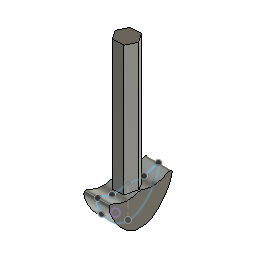
horse_support (Autodesk Fusion 360 design; units mm, degrees)
part number: 2026-05-20-21-49-29-160
Autodesk Fusion 360 part; units mm, degrees
derive "DerivedContext1"
sketch "Sketch1" plane through (0, 0, 0) normal (1, 0, 0) x (0, 1, 0)
  line L0 (-161.6595, 88.3093) -> (-161.6595, 78.1224)
  spline S0 degree 5 poles (-161.6595, 88.3093) (-161.5029, 88.2799) (-161.1728, 88.2083) (-160.6272, 88.0626) (-159.8017, 87.8168) (-158.6304, 87.5525) (-157.3592, 87.4678) (-156.0437, 87.6541) (-154.7574, 88.0873) (-153.5882, 88.6143) (-152.6243, 89.0285) (-151.9436, 89.1235) (-151.601, 88.7551) (-151.6157, 87.9035) (-151.9774, 86.6432) (-152.6539, 85.1075) (-153.5977, 83.4578) (-154.7519, 81.8484) (-156.0558, 80.4054) (-157.4494, 79.2317) (-158.8779, 78.4066) (-160.0123, 78.0714) (-160.8446, 78.0183) (-161.3895, 78.0728) (-161.6595, 78.1224) knots 0 0 0 0 0 0 0.05 0.1 0.15 0.2 0.25 0.3 0.35 0.4 0.45 0.5 0.55 0.6 0.65 0.7 0.75 0.8 0.85 0.9 0.95 1 1 1 1 1 1
  line L1 (-165.3917, 89.0107) -> (-157.9274, 87.6079)
  line L2 (-157.7822, 77.4094) -> (-165.5368, 78.8354)
  spline S1 degree 5 poles (-161.6595, 88.3093) (-161.8161, 88.2799) (-162.1462, 88.2083) (-162.6919, 88.0626) (-163.5173, 87.8168) (-164.6886, 87.5525) (-165.9599, 87.4678) (-167.2754, 87.6541) (-168.5616, 88.0873) (-169.7309, 88.6143) (-170.6948, 89.0285) (-171.3755, 89.1235) (-171.718, 88.7551) (-171.7033, 87.9035) (-171.3417, 86.6432) (-170.6652, 85.1075) (-169.7214, 83.4578) (-168.5671, 81.8484) (-167.2632, 80.4054) (-165.8696, 79.2317) (-164.4412, 78.4066) (-163.3067, 78.0714) (-162.4745, 78.0183) (-161.9295, 78.0728) (-161.6595, 78.1224) knots 0 0 0 0 0 0 0.05 0.1 0.15 0.2 0.25 0.3 0.35 0.4 0.45 0.5 0.55 0.6 0.65 0.7 0.75 0.8 0.85 0.9 0.95 1 1 1 1 1 1
  line L3 (-157.9274, 89.0107) -> (-165.3917, 87.6079)
  line L4 (-165.5368, 77.4094) -> (-157.7822, 78.8354)
  point P0 (-156.5652, 87.6135)
  point P1 (-152, 89)
  point P2 (-153.319, 84)
  point P3 (-166.7538, 87.6135)
  point P4 (-171.319, 89)
  point P5 (-170, 84)
  constraint vertical L0
  constraint coincident L0 S0.end
  constraint midpoint L0.start L1
  constraint midpoint L0.end L2
  constraint symmetric P0 L0 P3
  constraint symmetric P1 L0 P4
  constraint symmetric P2 L0 P5
  constraint symmetric L0 S0.start S1.start
  constraint symmetric L0 S0.end S1.end
  constraint symmetric L0 L1.start L3.start
  constraint symmetric L0 L1.end L3.end
  constraint symmetric L0 L2.start L4.start
  constraint symmetric L0 L2.end L4.end
extrude "Extrude1" add sketch "Sketch1" along normal mid plane 8
sketch "Sketch2" plane through (-4, 0, 0) normal (-1, 0, 0) x (0, -1, 0)
  spline S0 degree 5 poles (161.6595, 78.1224) (161.9295, 78.0728) (162.4745, 78.0183) (163.3067, 78.0714) (164.4412, 78.4066) (165.8696, 79.2317) (167.2632, 80.4054) (168.5671, 81.8484) (169.7214, 83.4578) (170.6652, 85.1075) (171.3417, 86.6432) (171.7033, 87.9035) (171.718, 88.7551) (171.3755, 89.1235) (170.6948, 89.0285) (169.7309, 88.6143) (168.5616, 88.0873) (167.2754, 87.6541) (165.9599, 87.4678) (164.6886, 87.5525) (163.5173, 87.8168) (162.6919, 88.0626) (162.1462, 88.2083) (161.8161, 88.2799) (161.6595, 88.3093) knots -1 -1 -1 -1 -1 -1 -0.95 -0.9 -0.85 -0.8 -0.75 -0.7 -0.65 -0.6 -0.55 -0.5 -0.45 -0.4 -0.35 -0.3 -0.25 -0.2 -0.15 -0.1 -0.05 0 0 0 0 0 0
  spline S1 degree 5 poles (161.6595, 88.3093) (161.5029, 88.2799) (161.1728, 88.2083) (160.6272, 88.0626) (159.8017, 87.8168) (158.6304, 87.5525) (157.3592, 87.4678) (156.0437, 87.6541) (154.7574, 88.0873) (153.5882, 88.6143) (152.6243, 89.0285) (151.9436, 89.1235) (151.601, 88.7551) (151.6157, 87.9035) (151.9774, 86.6432) (152.6539, 85.1075) (153.5977, 83.4578) (154.7519, 81.8484) (156.0558, 80.4054) (157.4494, 79.2317) (158.8779, 78.4066) (160.0123, 78.0714) (160.8446, 78.0183) (161.3895, 78.0728) (161.6595, 78.1224) knots 0 0 0 0 0 0 0.05 0.1 0.15 0.2 0.25 0.3 0.35 0.4 0.45 0.5 0.55 0.6 0.65 0.7 0.75 0.8 0.85 0.9 0.95 1 1 1 1 1 1
ref_plane "WorkPlane1" through (-4, -160.339, 88.8588) normal (0, 0, 1) x (-1, 0, 0)
sketch "Sketch3" plane through (0, 0, 88.8588) normal (0, 0, 1) x (1, 0, 0)
  line L0 (1.9423, -164.9116) -> (3.4927, -161.7737)
  line L1 (3.4927, -161.7737) -> (1.5503, -158.8621)
  line L2 (1.5503, -158.8621) -> (-1.9423, -159.0884)
  line L3 (-1.9423, -159.0884) -> (-3.4927, -162.2263)
  line L4 (-3.4927, -162.2263) -> (-1.5503, -165.1379)
  line L5 (-1.5503, -165.1379) -> (1.9423, -164.9116)
  point P0 (0, -162)
  dimension "d4" = 3.5
  measures "d4" distance of L0.start P0
extrude "Extrude2" add sketch "Sketch3" along normal blind 40 and the other way blind 1.5
